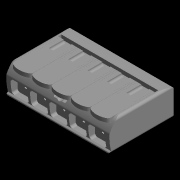
# Autodesk Inventor part: 221-415
Saved by Autodesk Inventor 2020.2 (Build 242310000, 310)
## iProperties
Part Number: 221-415
Material: Generic
Catalog Web Link: www.cadenas.de
Description: 221-415-COMPACT splicing connectors for all conductor types 5-conductor terminal block
Vendor: WAGO
Document SubType Name: Modeling
Designer: partserver
Manufacturer: WAGO
Mass: 4.048 g
Surface Area: 25.6811 cm^2
Volume: 4.16397 cm^3
Density: 1 g/cm^3
Appearance: PSOLRGB-175-175-175
Category: PARTsolutions
Company: WAGO
PSOL_IDENT_0: {$CADENAS_DATA\23d-libs\wago\pg07\serie221\0221-0415_0999-0962.prj},155 {VTYP=3D},{NB=221-415},{LINA=
PSOL_IDENT_1: 221-415},{NN=221-415},{DATE=29.01.2020 12:06:42},{GEOMDATE=25.10.2019 05:45:11},{VERSION=},{LINEID=2
PSOL_IDENT_2: 0},{WBVAR=},{WBNUMERIC=}  {NB=221-415},{LINA=221-415},{KT=DUMMY},{BESTNR=221-415},{INFODE=Info DE},{
PSOL_IDENT_3: INFOEN=Info EN},{QUERSCHNITT1=0.2 - 4 \"e + m\"  /  0.14 - 4 \"f\"},{QUERSCHNITT2=24 - 12},{ABISOLIE
PSOL_IDENT_4: RLAENGE=11},{SPANNUNG=450},{BEMESSSTOSSSPG=4},{VERSCHMUTZGRAD=2},{STROM=32},{P=5},{HOEHE=8.30},{BREI
PSOL_IDENT_5: TE=29.90},{TIEFE=18.60},{ANZAHLKLEMMSTEL=5},{ANZAHLPOTENTIAL=5},{FARBE=transparent},{GEWICHT=4.048},
PSOL_IDENT_6: {LINKDE=http://www.wago.com/de/p/221-415},{LINKEN=http://www.wago.com/global/p/221-415}
NB: 221-415
NN: 221-415
NT: COMPACT splicing connectors for all conductor types 5-conductor terminal block
NBSYN: $BESTNR.
LINA: 221-415
CATALOG: WAGO
OFFICIAL_STANDARD_NUMBERS: NO
BESTNR: 221-415
INFODE: Info DE
INFOEN: Info EN
QUERSCHNITT1: 0.2 - 4 "e + m"  /  0.14 - 4 "f"
QUERSCHNITT2: 24 - 12
ABISOLIERLAENGE: 11
SPANNUNG: 450
BEMESSSTOSSSPG: 4
VERSCHMUTZGRAD: 2
STROM: 32
P: 5
HOEHE: 8.3
BREITE: 29.9
TIEFE: 18.6
ANZAHLKLEMMSTEL: 5
ANZAHLPOTENTIAL: 5
FARBE: transparent
GEWICHT: 4.048
SUPPLIER: WAGO
ARTICLENO: 221-415
BOMINFO: 221-415
CREATOR: CADENAS GmbH
Title: 221-415
Author: Cadenas PARTsolutions
Comments: COMPACT splicing connectors for all conductor types 5-conductor terminal block
Autodesk Inventor part; units mm, degrees
ref_plane "YZ Plane" through (0, 0, 0) normal (1, 0, 0) x (0, 1, 0)
ref_plane "XZ Plane" through (0, 0, 0) normal (0, 1, 0) x (-1, 0, 0)
ref_plane "XY Plane" through (0, 0, 0) normal (0, 0, 1) x (1, 0, 0)
sketch "Sketch_1" plane through (0, 0, 0) normal (0, 0, 1) x (1, 0, 0)
  line L0 (0, 7.2187) -> (0, 0)
  line L1 (0, 0) -> (18.4, 0)
  arc A0 (18.4, 0) -> (18.6, 0.2) centre (18.4, 0.2) ccw
  line L2 (18.6, 0.2) -> (18.6, 0.2905)
  arc A1 (18.6, 0.2905) -> (18.4845, 0.4717) centre (18.4, 0.2905) ccw
  line L3 (18.4845, 0.4717) -> (18.1022, 0.65)
  arc A2 (18.1022, 0.65) -> (18.5749, 4.9468) centre (4.69, 4.3) ccw
  arc A3 (18.5749, 4.9468) -> (18.4726, 5.3431) centre (17.576, 4.9002) ccw
  arc A4 (18.4726, 5.3431) -> (17.0892, 7.3213) centre (11.3, 1.8) ccw
  arc A5 (17.0892, 7.3213) -> (15.23, 8.15) centre (15.23, 5.65) ccw
  line L4 (15.23, 8.15) -> (3.62, 8.15)
  arc A6 (3.62, 8.15) -> (0.3643, 7.6999) centre (3.62, -3.85) ccw
  arc A7 (0.3643, 7.6999) -> (0, 7.2187) centre (0.5, 7.2187) ccw
  constraints: 16 point on circle, 10 end point, 8 centre point
extrude "Extrusion1" add sketch "Sketch_1" along normal blind 29.8
sketch "Sketch_5" plane through (0, 0, 0) normal (1, 0, 0) x (0, 1, 0)
  line L0 (9.15, 30.8) -> (-1, 30.8)
  line L1 (-1, 30.8) -> (-1, -1)
  line L2 (-1, -1) -> (9.15, -1)
  line L3 (9.15, -1) -> (9.15, 30.8)
  line L4 (7.45, 29.8) -> (0.7, 29.8)
  arc A0 (0.7, 29.8) -> (0, 29.1) centre (0.7, 29.1) ccw
  line L5 (0, 29.1) -> (0, 0.7)
  arc A1 (0, 0.7) -> (0.7, 0) centre (0.7, 0.7) ccw
  line L6 (0.7, 0) -> (7.45, 0)
  arc A2 (7.45, 0) -> (8.15, 0.7) centre (7.45, 0.7) ccw
  line L7 (8.15, 0.7) -> (8.15, 29.1)
  arc A3 (8.15, 29.1) -> (7.45, 29.8) centre (7.45, 29.1) ccw
  constraints: 16 end point, 8 point on circle, 4 centre point
extrude "Extrusion2" cut sketch "Sketch_5" along normal blind 18.6
sketch "Sketch_2" plane through (18.6, 0, 0) normal (1, 0, 0) x (0, 0, -1)
  line L0 (-6.15, 4.07) -> (-6.15, 1.35)
  arc A0 (-6.15, 1.35) -> (-5.45, 0.65) centre (-5.45, 1.35) ccw
  line L1 (-5.45, 0.65) -> (-1.95, 0.65)
  arc A1 (-1.95, 0.65) -> (-1.25, 1.35) centre (-1.95, 1.35) ccw
  line L2 (-1.25, 1.35) -> (-1.25, 4.07)
  arc A2 (-1.25, 4.07) -> (-1.95, 4.77) centre (-1.95, 4.07) ccw
  line L3 (-1.95, 4.77) -> (-5.45, 4.77)
  arc A3 (-5.45, 4.77) -> (-6.15, 4.07) centre (-5.45, 4.07) ccw
  constraints: 8 end point, 8 point on circle, 4 centre point
extrude "Extrusion3" cut sketch "Sketch_2" against normal blind 2
pattern_linear "Rectangular Pattern1" count 5 spacing 5.6 along (0, 0, 1) of "Extrusion3"
sketch "Sketch_4" plane through (18.6, 0, 0) normal (1, 0, 0) x (0, 0, -1)
  line L0 (-16.675, 7.3) -> (-16.675, 6.3)
  arc A0 (-16.675, 6.3) -> (-16.375, 6) centre (-16.375, 6.3) ccw
  line L1 (-16.375, 6) -> (-15.5408, 6)
  arc A1 (-15.5408, 6) -> (-14.2592, 6) centre (-14.9, 6.8) ccw
  line L2 (-14.2592, 6) -> (-13.425, 6)
  arc A2 (-13.425, 6) -> (-13.125, 6.3) centre (-13.425, 6.3) ccw
  line L3 (-13.125, 6.3) -> (-13.125, 7.3)
  arc A3 (-13.125, 7.3) -> (-13.425, 7.6) centre (-13.425, 7.3) ccw
  line L4 (-13.425, 7.6) -> (-14.2592, 7.6)
  arc A4 (-14.2592, 7.6) -> (-15.5408, 7.6) centre (-14.9, 6.8) ccw
  line L5 (-15.5408, 7.6) -> (-16.375, 7.6)
  arc A5 (-16.375, 7.6) -> (-16.675, 7.3) centre (-16.375, 7.3) ccw
  constraints: 12 end point, 12 point on circle, 6 centre point
extrude "Extrusion4" cut sketch "Sketch_4" against normal blind 2
sketch "Sketch_6" plane through (18.6, 0, 0) normal (1, 0, 0) x (0, 0, -1)
  line L0 (-6.5, 7) -> (-5.96, 7)
  line L1 (-5.96, 7) -> (-5.96, 8.15)
  line L2 (-5.96, 8.15) -> (-1.44, 8.15)
  line L3 (-1.44, 8.15) -> (-1.44, 7)
  line L4 (-1.44, 7) -> (-0.9, 7)
  line L5 (-0.9, 7) -> (-0.9, 9.15)
  line L6 (-0.9, 9.15) -> (-6.5, 9.15)
  line L7 (-6.5, 9.15) -> (-6.5, 7)
  constraints: 16 end point
extrude "Extrusion5" cut sketch "Sketch_6" against normal blind 14.98
pattern_linear "Rectangular Pattern2" count 3 spacing 11.2 along (0, 0, 1) of "Extrusion5"
sketch "Sketch_13" plane through (18.6, 0, 0) normal (1, 0, 0) x (0, 0, -1)
  line L0 (-12.1, 7) -> (-11.56, 7)
  line L1 (-11.56, 7) -> (-11.56, 8.15)
  line L2 (-11.56, 8.15) -> (-7.04, 8.15)
  line L3 (-7.04, 8.15) -> (-7.04, 7)
  line L4 (-7.04, 7) -> (-6.5, 7)
  line L5 (-6.5, 7) -> (-6.5, 9.15)
  line L6 (-6.5, 9.15) -> (-12.1, 9.15)
  line L7 (-12.1, 9.15) -> (-12.1, 7)
  constraints: 16 end point
extrude "Extrusion6" cut sketch "Sketch_13" against normal blind 14.98
pattern_linear "Rectangular Pattern3" count 2 spacing 11.2 along (0, 0, 1) of "Extrusion6"
sketch "Sketch_8" plane through (0, 8.15, 0) normal (0, 1, 0) x (1, 0, 0)
  line L0 (4.55, -5.98) -> (4.55, -6.48)
  line L1 (4.55, -6.48) -> (17.1821, -6.48)
  arc A0 (17.1821, -6.48) -> (18.0777, -5.925) centre (17.1821, -5.48) ccw
  arc A1 (18.0777, -5.925) -> (18.0777, -1.475) centre (13.6, -3.7) ccw
  arc A2 (18.0777, -1.475) -> (17.1821, -0.92) centre (17.1821, -1.92) ccw
  line L2 (17.1821, -0.92) -> (4.55, -0.92)
  line L3 (4.55, -0.92) -> (4.55, -1.42)
  line L4 (4.55, -1.42) -> (10.25, -1.42)
  arc A3 (10.65, -1.82) -> (10.25, -1.42) centre (10.25, -1.82) ccw
  line L5 (10.65, -1.82) -> (10.65, -5.58)
  arc A4 (10.25, -5.98) -> (10.65, -5.58) centre (10.25, -5.58) ccw
  line L6 (10.25, -5.98) -> (4.55, -5.98)
  constraints: 14 end point, 10 point on circle, 5 centre point
extrude "Extrusion7" add sketch "Sketch_8" against normal blind 1.1
pattern_linear "Rectangular Pattern4" count 5 spacing 5.6 along (0, 0, 1) of "Extrusion7"
sketch "Sketch_10" plane through (3.62, 0, 0) normal (1, 0, 0) x (0, 0, -1)
  arc A0 (-4.86, 8) -> (-4.26, 7.4) centre (-4.26, 8) ccw
  line L0 (-4.26, 7.4) -> (-3.14, 7.4)
  arc A1 (-3.14, 7.4) -> (-2.54, 8) centre (-3.14, 8) ccw
  line L1 (-2.54, 8) -> (-2.54, 8.15)
  line L2 (-2.54, 8.15) -> (-4.86, 8.15)
  line L3 (-4.86, 8.15) -> (-4.86, 8)
  constraints: 8 end point, 4 point on circle, 2 centre point
extrude "Extrusion8" cut sketch "Sketch_10" along normal blind 5.2
pattern_linear "Rectangular Pattern5" count 5 spacing 5.6 along (0, 0, 1) of "Extrusion8"
sketch "Sketch_12" plane through (0, 0, 0.9) normal (0, 0, 1) x (1, 0, 0)
  line L0 (3.62, 7) -> (4.55, 7)
  line L1 (4.55, 7) -> (4.55, 8.15)
  line L2 (4.55, 8.15) -> (3.62, 8.15)
  line L3 (3.62, 8.15) -> (3.62, 7)
  constraints: 8 end point
extrude "Extrusion9" cut sketch "Sketch_12" along normal blind 28
sketch "Sketch10" plane through (16.6, 1.35, 28.55) normal (1, 0, 0) x (0, 0, -1)
  line L0 (0, 0) -> (0, 2.72) construction
  arc A0 (0, 0) -> (0.7, -0.7) centre (0.7, 0) ccw construction
  line L1 (4.2, -0.7) -> (0.7, -0.7) construction
  arc A1 (4.2, -0.7) -> (4.9, 0) centre (4.2, 0) ccw construction
  line L2 (4.9, 2.72) -> (4.9, 0) construction
  arc A2 (4.9, 2.72) -> (4.2, 3.42) centre (4.2, 2.72) ccw construction
  line L3 (0.7, 3.42) -> (4.2, 3.42) construction
  arc A3 (0.7, 3.42) -> (0, 2.72) centre (0.7, 2.72) ccw construction
  line L4 (5.6, 0) -> (5.6, 2.72) construction
  arc A4 (5.6, 0) -> (6.3, -0.7) centre (6.3, 0) ccw construction
  line L5 (9.8, -0.7) -> (6.3, -0.7) construction
  arc A5 (9.8, -0.7) -> (10.5, 0) centre (9.8, 0) ccw construction
  line L6 (10.5, 2.72) -> (10.5, 0) construction
  arc A6 (10.5, 2.72) -> (9.8, 3.42) centre (9.8, 2.72) ccw construction
  line L7 (6.3, 3.42) -> (9.8, 3.42) construction
  arc A7 (6.3, 3.42) -> (5.6, 2.72) centre (6.3, 2.72) ccw construction
  line L8 (11.2, 0) -> (11.2, 2.72) construction
  arc A8 (11.2, 0) -> (11.9, -0.7) centre (11.9, 0) ccw construction
  line L9 (15.4, -0.7) -> (11.9, -0.7) construction
  arc A9 (15.4, -0.7) -> (16.1, 0) centre (15.4, 0) ccw construction
  line L10 (16.1, 2.72) -> (16.1, 0) construction
  arc A10 (16.1, 2.72) -> (15.4, 3.42) centre (15.4, 2.72) ccw construction
  line L11 (11.9, 3.42) -> (15.4, 3.42) construction
  arc A11 (11.9, 3.42) -> (11.2, 2.72) centre (11.9, 2.72) ccw construction
  line L12 (16.8, 0) -> (16.8, 2.72) construction
  arc A12 (16.8, 0) -> (17.5, -0.7) centre (17.5, 0) ccw construction
  line L13 (21, -0.7) -> (17.5, -0.7) construction
  arc A13 (21, -0.7) -> (21.7, 0) centre (21, 0) ccw construction
  line L14 (21.7, 2.72) -> (21.7, 0) construction
  arc A14 (21.7, 2.72) -> (21, 3.42) centre (21, 2.72) ccw construction
  line L15 (17.5, 3.42) -> (21, 3.42) construction
  arc A15 (17.5, 3.42) -> (16.8, 2.72) centre (17.5, 2.72) ccw construction
  line L16 (22.4, 0) -> (22.4, 2.72) construction
  arc A16 (22.4, 0) -> (23.1, -0.7) centre (23.1, 0) ccw construction
  line L17 (26.6, -0.7) -> (23.1, -0.7) construction
  arc A17 (26.6, -0.7) -> (27.3, 0) centre (26.6, 0) ccw construction
  line L18 (27.3, 2.72) -> (27.3, 0) construction
  arc A18 (27.3, 2.72) -> (26.6, 3.42) centre (26.6, 2.72) ccw construction
  line L19 (23.1, 3.42) -> (26.6, 3.42) construction
  arc A19 (23.1, 3.42) -> (22.4, 2.72) centre (23.1, 2.72) ccw construction
  line L20 (0.7, 2.72) -> (4.2, 0) construction
  line L21 (6.3, 2.72) -> (9.8, 0) construction
  line L22 (11.9, 2.72) -> (15.4, 0) construction
  line L23 (17.5, 2.72) -> (21, 0) construction
  line L24 (23.1, 2.72) -> (26.6, 0) construction
  point P0 (28.55, -1.35)
  point P1 (24.85, 1.36)
  point P2 (19.25, 1.36)
  point P3 (13.65, 1.36)
  point P4 (8.05, 1.36)
  point P5 (2.45, 1.36)
  constraints: 10 end point, 5 midpoint, 3 parallel
body "Solid1"
